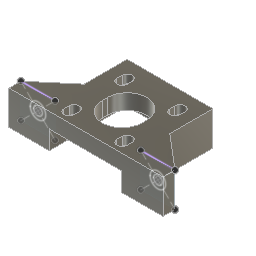
Z Axis Motor Mount (Autodesk Fusion 360 design; units mm, degrees)
Autodesk Fusion 360 part; units mm, degrees
sketch "Sketch1" plane through (0, 0, 0) normal (0, 0, 1) x (1, 0, 0)
  line L0 (45.1, -24.6) -> (-45.1, -24.6)
  line L1 (-45.1, -24.6) -> (-45.1, 24.6)
  line L2 (-45.1, 24.6) -> (45.1, 24.6)
  line L3 (45.1, 24.6) -> (45.1, -24.6)
  line L4 (45.1, -24.6) -> (-45.1, 24.6) construction
  line L5 (-45.1, -24.6) -> (45.1, 24.6) construction
  dimension "d1" = 90.2
  dimension "d2" = 49.2
  constraint perpendicular L0 L1
  constraint parallel L0 L2
  constraint parallel L1 L3
  constraint horizontal L0
  constraint coincident L4 origin
  constraint coincident L5 origin
  measures "d1" distance of L1.end L2.end
  measures "d2" distance of L0.end L1.end L0.start
  measures "d5" distance of L0.start
extrude "Extrude1" add sketch "Sketch1" along normal blind 20
sketch "Sketch2" plane through (0, 0, 0) normal (0, 0, -1) x (-1, 0, 0)
  line L0 (40.1, -22.1) -> (40.1, 22.1)
  line L1 (40.1, 22.1) -> (-40.1, 22.1)
  line L2 (-40.1, 22.1) -> (-40.1, -22.1)
  line L3 (21.4974, -24.6) -> (-20.7026, -24.6)
  line L4 (-20.7026, -24.6) -> (-20.7026, 20.6)
  line L5 (-20.7026, 20.6) -> (21.4974, 20.6)
  line L6 (21.4974, 20.6) -> (21.4974, -24.6)
  line L7 (45.1, 24.6) -> (-45.1, 24.6)
  line L8 (-45.1, 24.6) -> (-45.1, -24.6)
  line L9 (-45.1, -24.6) -> (45.1, -24.6)
  line L10 (45.1, -24.6) -> (45.1, 24.6)
  dimension "d5" = 42.2
  dimension "d6" = 45.2
  constraint horizontal L3
  constraint vertical L4
  constraint horizontal L5
  constraint vertical L6
  constraint coincident L3.start L9
  measures "d5" distance of L3.start L3.end
  measures "d6" distance of L3.start L5.end
extrude "Extrude2" cut sketch "Sketch2" against normal blind 11 contours L3 L4 L5 L6 L9
sketch "Sketch3" plane through (0, 24.6, 0) normal (0, 1, 0) x (-1, 0, 0)
  line L0 (-45.1, 0) -> (45.1, 0)
  line L1 (45.1, 0) -> (45.1, 20)
  line L2 (45.1, 20) -> (-45.1, 20)
  line L3 (-45.1, 20) -> (-45.1, 0)
  line L4 (-45.1, 20) -> (-25.1, 20)
  line L5 (-25.1, 20) -> (-25.1, 0)
  line L6 (-25.1, 0) -> (-45.1, 0)
  line L7 (-45.1, 0) -> (-45.1, 20)
  line L8 (45.1, 20) -> (25.1, 20)
  line L9 (25.1, 20) -> (25.1, 0)
  line L10 (25.1, 0) -> (45.1, 0)
  line L11 (45.1, 0) -> (45.1, 20)
  dimension "d9" = 20
  dimension "d10" = 20
  constraint horizontal L4
  constraint vertical L5
  constraint horizontal L6
  constraint vertical L7
  constraint coincident L2.end L3.start
  constraint horizontal L8
  constraint vertical L9
  constraint horizontal L10
  constraint vertical L11
  constraint coincident L1.end L2.start
  measures "d9" distance of L2.end L4.end
  measures "d10" distance of L1.end L8.end
extrude "Extrude3" cut sketch "Sketch3" against normal blind 42.2 contours L0 L2 L3 L4 L5 L6 L7 | L0 L1 L2 L8 L9 L10 L11
sketch "Sketch4" plane through (0, 0, 20) normal (0, 0, 1) x (-1, 0, 0)
  line L0 (25.1, -24.6) -> (25.1, 17.6)
  line L1 (25.1, 17.6) -> (45.1, 17.6)
  line L2 (45.1, 17.6) -> (45.1, 24.6)
  line L3 (45.1, 24.6) -> (-45.1, 24.6)
  line L4 (-45.1, 24.6) -> (-45.1, 17.6)
  line L5 (-45.1, 17.6) -> (-25.1, 17.6)
  line L6 (-25.1, 17.6) -> (-25.1, -24.6)
  line L7 (-25.1, -24.6) -> (25.1, -24.6)
  line L8 (25.1, -13.5) -> (-25.1, -13.5) construction
  line L9 (-25.1, 17.5) -> (25.1, 17.5) construction
  line L10 (25.1, 16) -> (-25.1, 16) construction
  line L11 (25.1, 19) -> (-25.1, 19) construction
  line L12 (25.1, -12) -> (-25.1, -12) construction
  line L13 (-25.1, -15) -> (25.1, -15) construction
  line L14 (15.5, -24.6) -> (15.5, 19) construction
  line L15 (-15.5, -24.6) -> (-15.5, 19) construction
  line L16 (14, -12) -> (14, -15)
  arc A0 (14, -15) -> (17, -15) centre (15.5, -15) ccw
  line L17 (17, -15) -> (17, -12)
  arc A1 (17, -12) -> (14, -12) centre (15.5, -12) ccw
  line L18 (15.5, -12) -> (15.5, -15) construction
  line L19 (12.5, -12) -> (12.5, -15)
  arc A2 (12.5, -15) -> (18.5, -15) centre (15.5, -15) ccw
  line L20 (18.5, -15) -> (18.5, -12)
  arc A3 (18.5, -12) -> (12.5, -12) centre (15.5, -12) ccw
  line L21 (15.5, -12) -> (15.5, -15) construction
  line L22 (0, -24.6) -> (0, 24.6) construction
  line L23 (-25.1, 2) -> (25.1, 2) construction
  arc A4 (-14, -12) -> (-17, -12) centre (-15.5, -12) ccw
  line L24 (-14, -12) -> (-14, -15)
  arc A5 (-17, -15) -> (-14, -15) centre (-15.5, -15) ccw
  line L25 (-17, -15) -> (-17, -12)
  arc A6 (-12.5, -12) -> (-18.5, -12) centre (-15.5, -12) ccw
  line L26 (-12.5, -12) -> (-12.5, -15)
  line L27 (-18.5, -15) -> (-18.5, -12)
  arc A7 (-18.5, -15) -> (-12.5, -15) centre (-15.5, -15) ccw
  arc A8 (18.5, 19) -> (12.5, 19) centre (15.5, 19) ccw
  line L28 (18.5, 19) -> (18.5, 16)
  arc A9 (12.5, 16) -> (18.5, 16) centre (15.5, 16) ccw
  line L29 (12.5, 16) -> (12.5, 19)
  line L30 (17, 19) -> (17, 16)
  arc A10 (14, 16) -> (17, 16) centre (15.5, 16) ccw
  arc A11 (17, 19) -> (14, 19) centre (15.5, 19) ccw
  line L31 (14, 16) -> (14, 19)
  arc A12 (-14, 19) -> (-17, 19) centre (-15.5, 19) ccw
  line L32 (-17, 19) -> (-17, 16)
  arc A13 (-17, 16) -> (-14, 16) centre (-15.5, 16) ccw
  line L33 (-14, 16) -> (-14, 19)
  line L34 (-18.5, 19) -> (-18.5, 16)
  arc A14 (-12.5, 19) -> (-18.5, 19) centre (-15.5, 19) ccw
  line L35 (-12.5, 16) -> (-12.5, 19)
  arc A15 (-18.5, 16) -> (-12.5, 16) centre (-15.5, 16) ccw
  dimension "d13" = 31
  dimension "d14" = 7.1
  dimension "d55" = 1.5
  dimension "d56" = 1.5
  dimension "d57" = 1.5
  dimension "d58" = 1.5
  dimension "d59" = 9.6
  dimension "d60" = 9.6
  dimension "d61" = 3
  dimension "d62" = 6
  dimension "d63" = 15.5
  constraint coincident L0 L8.start
  constraint coincident L6 L8.end
  constraint perpendicular L6 L8
  constraint coincident L6 L9.start
  constraint coincident L0 L9.end
  constraint perpendicular L0 L9
  constraint coincident L0 L10.start
  constraint coincident L6 L10.end
  constraint perpendicular L6 L10
  constraint coincident L0 L11.start
  constraint coincident L6 L11.end
  constraint perpendicular L6 L11
  constraint coincident L0 L12.start
  constraint coincident L6 L12.end
  constraint perpendicular L6 L12
  constraint coincident L6 L13.start
  constraint coincident L0 L13.end
  constraint perpendicular L0 L13
  constraint coincident L7 L14.start
  constraint coincident L11 L14.end
  constraint perpendicular L11 L14
  constraint coincident L7 L15.start
  constraint coincident L11 L15.end
  constraint perpendicular L11 L15
  constraint tangent L16 A0
  constraint tangent A0 L17
  constraint parallel L16 L17
  constraint tangent L17 A1
  constraint tangent L16 A1
  constraint coincident L14 A0.centre
  constraint coincident L13 A0.centre
  constraint perpendicular L13 L18
  constraint coincident L12 A1.centre
  constraint tangent L19 A2
  constraint tangent A2 L20
  constraint parallel L19 L20
  constraint tangent L20 A3
  constraint tangent L19 A3
  constraint coincident A0.centre L18.end
  constraint perpendicular L13 L21
  constraint coincident A1.centre L18.start
  constraint midpoint L7 L22.start
  constraint midpoint L3 L22.end
  constraint coincident L6 L23.start
  constraint coincident L0 L23.end
  constraint perpendicular L0 L23
  constraint symmetric L16.start L22 A4.start
  constraint symmetric L16.end L22 L24.end
  constraint symmetric A0.end L22 A5.start
  constraint symmetric L17.end L22 A4.end
  constraint symmetric A0 L22 A5
  constraint symmetric A1 L22 A4
  constraint symmetric L19.start L22 A6.start
  constraint symmetric L19.end L22 L26.end
  constraint symmetric A2.end L22 L27.start
  constraint symmetric L20.end L22 A6.end
  constraint symmetric A2 L22 A7
  constraint symmetric A3 L22 A6
  constraint symmetric L16.start L23 A10.start
  constraint symmetric L16.end L23 A11.end
  constraint symmetric A0.end L23 L30.start
  constraint symmetric L17.end L23 L30.end
  constraint symmetric A0 L23 A11
  constraint symmetric A1 L23 A10
  constraint symmetric L19.start L23 A9.start
  constraint symmetric L19.end L23 A8.end
  constraint symmetric A2.end L23 A8.start
  constraint symmetric L20.end L23 L28.end
  constraint symmetric A2 L23 A8
  constraint symmetric A3 L23 A9
  constraint symmetric L23 A4.end L32.end
  constraint symmetric L23 A4.start A13.end
  constraint symmetric L23 A4 A13
  constraint symmetric L23 L24.end A12.start
  constraint symmetric L23 A5.start A12.end
  constraint symmetric L23 A5 A12
  constraint symmetric L23 A6.end L34.end
  constraint symmetric L23 A6.start L35.start
  constraint symmetric L23 A6 A15
  constraint symmetric L23 L26.end A14.start
  constraint symmetric L23 L27.start L34.start
  constraint symmetric L23 A7 A14
  measures "d13" distance of L8 L9
  measures "d14" distance of L3 L9
  measures "d55" distance of L8 L13
  measures "d56" distance of L8 L12
  measures "d57" distance of L9 L10
  measures "d58" distance of L9 L11
  measures "d59" distance of L6 L15
  measures "d60" distance of L0 L14
  measures "d61" diameter of A0
  measures "d62" diameter of A2
  measures "d63" distance of L8 L23
extrude "Extrude5" cut sketch "Sketch4" against normal blind 5 contours L16 A0 L17 A1 | L19 A2 L20 A3 | A4 L24 A5 L25 | A6 L26 L27 A7 | A8 L28 A9 L29 | L30 A10 A11 L31 | A12 L32 A13 L33 | L34 A14 L35 A15
extrude "Extrude4" cut sketch "Sketch4" against normal blind 9 from surface at -5.2 contours L16 A0 L17 A1 | A4 L24 A5 L25 | L30 A10 A11 L31 | A12 L32 A13 L33
sketch "Sketch5" plane through (0, -17.6, 0) normal (0, 1, 0) x (-1, 0, 0)
  line L0 (-45.1, 20) -> (-45.1, 0)
  line L1 (-45.1, 0) -> (-25.1, 0)
  line L2 (-25.1, 0) -> (-25.1, 20)
  line L3 (-25.1, 20) -> (-45.1, 0) construction
  line L4 (-45.1, 20) -> (-25.1, 0) construction
  circle A0 centre (-35.1, 10) radius 2.5
  circle A1 centre (-35.1, 10) radius 4.5
  line L5 (-25.1, 20) -> (-45.1, 20)
  dimension "d33" = 5
  dimension "d34" = 9
  constraint coincident L2.end L3.start
  constraint coincident L0.end L1.start
  constraint coincident L0.start L4.start
  constraint coincident L1.end L2.start
  constraint midpoint L3 A0.centre
  constraint concentric A0 A1
  measures "d33" diameter of A0
  measures "d34" diameter of A1
extrude "Extrude8" cut sketch "Sketch5" against normal blind 1 contours A0 | A1
extrude "Extrude7" cut sketch "Sketch5" against normal blind 4 contours A0
sketch "Sketch6" plane through (0, -17.6, 0) normal (0, 1, 0) x (-1, 0, 0)
  line L0 (45.1, 0) -> (45.1, 20)
  line L1 (25.1, 20) -> (25.1, 0)
  line L2 (25.1, 0) -> (45.1, 0)
  line L3 (25.1, 0) -> (45.1, 20) construction
  line L4 (25.1, 20) -> (45.1, 0) construction
  circle A0 centre (35.1, 10) radius 2.5
  circle A1 centre (35.1, 10) radius 4.5
  line L5 (45.1, 20) -> (25.1, 20)
  point P0 (-12.5, -15)
  point P1 (-12.5, 19)
  dimension "d39" = 5
  dimension "d40" = 9
  constraint coincident L1.end L2.start
  constraint coincident L0.end L3.end
  constraint coincident L1.start L4.start
  constraint coincident L0.start L2.end
  constraint midpoint L4 A0.centre
  constraint concentric A0 A1
  measures "d39" diameter of A0
  measures "d40" diameter of A1
extrude "Extrude10" cut sketch "Sketch6" against normal blind 1 contours A0 | A1
extrude "Extrude9" cut sketch "Sketch6" against normal blind 4 contours A0
sketch "Sketch7" plane through (0, 0, 20) normal (0, 0, 1) x (-1, 0, 0)
  line L0 (25.1, -24.6) -> (25.1, 17.6)
  line L1 (25.1, 17.6) -> (45.1, 17.6)
  line L2 (45.1, 17.6) -> (45.1, 24.6)
  line L3 (45.1, 24.6) -> (-45.1, 24.6)
  line L4 (-45.1, 24.6) -> (-45.1, 17.6)
  line L5 (-45.1, 17.6) -> (-25.1, 17.6)
  line L6 (-25.1, 17.6) -> (-25.1, -24.6)
  line L7 (-25.1, -24.6) -> (25.1, -24.6)
  line L8 (-25.1, 0.6) -> (25.1, 0.6) construction
  line L9 (45.1, 24.6) -> (-45.1, 24.6) construction
  line L10 (45.1, 17.6) -> (25.1, 0.6)
  line L11 (-25.1, 0.6) -> (-45.1, 17.6)
  line L12 (15.5, -13.5) -> (-15.5, 17.5) construction
  line L13 (15.5, 17.5) -> (-15.5, -13.5) construction
  line L14 (-18.5, -15) -> (-18.5, -12)
  arc A0 (-12.5, -12) -> (-18.5, -12) centre (-15.5, -12) ccw
  line L15 (-12.5, -12) -> (-12.5, -15)
  arc A1 (-18.5, -15) -> (-12.5, -15) centre (-15.5, -15) ccw
  line L16 (12.5, -15) -> (12.5, -12)
  arc A2 (18.5, -12) -> (12.5, -12) centre (15.5, -12) ccw
  line L17 (18.5, -12) -> (18.5, -15)
  arc A3 (12.5, -15) -> (18.5, -15) centre (15.5, -15) ccw
  line L18 (-12.5, 19) -> (-12.5, 16)
  arc A4 (-18.5, 16) -> (-12.5, 16) centre (-15.5, 16) ccw
  line L19 (-18.5, 16) -> (-18.5, 19)
  arc A5 (-12.5, 19) -> (-18.5, 19) centre (-15.5, 19) ccw
  line L20 (12.5, 16) -> (12.5, 19)
  arc A6 (18.5, 19) -> (12.5, 19) centre (15.5, 19) ccw
  line L21 (18.5, 19) -> (18.5, 16)
  arc A7 (12.5, 16) -> (18.5, 16) centre (15.5, 16) ccw
  line L22 (25.1, 2) -> (-25.1, 2) construction
  line L23 (-25.1, 0.5) -> (25.1, 0.5) construction
  line L24 (25.1, 3.5) -> (-25.1, 3.5) construction
  line L25 (-11.5, 3.5) -> (-11.5, 0.5)
  arc A8 (-11.5, 0.5) -> (11.5, 0.5) centre (0, 0.5) ccw
  line L26 (11.5, 0.5) -> (11.5, 3.5)
  arc A9 (11.5, 3.5) -> (-11.5, 3.5) centre (0, 3.5) ccw
  line L27 (0, 3.5) -> (0, 0.5) construction
  dimension "d50" = 24
  dimension "d64" = 22.6
  dimension "d65" = 1.5
  dimension "d66" = 1.5
  dimension "d67" = 23
  constraint coincident L6 L8.start
  constraint coincident L0 L8.end
  constraint perpendicular L0 L8
  constraint coincident L1.end L2.start
  constraint coincident L4.end L5.start
  constraint coincident L0 L22.start
  constraint coincident L6 L22.end
  constraint perpendicular L6 L22
  constraint coincident L6 L23.start
  constraint coincident L0 L23.end
  constraint perpendicular L0 L23
  constraint coincident L0 L24.start
  constraint coincident L6 L24.end
  constraint perpendicular L6 L24
  constraint tangent L25 A8
  constraint tangent A8 L26
  constraint parallel L25 L26
  constraint tangent L26 A9
  constraint tangent L25 A9
  constraint perpendicular L23 L27
  constraint midpoint L24 A9.centre
  measures "d50" distance of L8 L9
  measures "d64" distance of L9 L22
  measures "d65" distance of L22 L23
  measures "d66" distance of L22 L24
  measures "d67" diameter of A8
extrude "Extrude13" cut sketch "Sketch7" against normal blind 9 contours L25 A8 L26 A9
extrude "Extrude11" add sketch "Sketch7" against normal blind 4 contours L0 L1 L10 | L5 L6 L11
extrude "Extrude12" add sketch "Sketch7" along normal blind 4 from surface at -20 contours L0 L1 L10 | L5 L6 L11
chamfer "Chamfer1" distance 4 angle 45 2 edges at (20.7026, 20.6, 5.5) (-21.4974, 20.6, 5.5)
